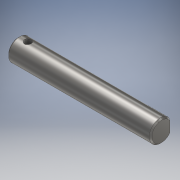
# Autodesk Inventor part: Crankshaft outer rod
Saved by Autodesk Inventor 2017 (Build 210142000, 142)
## iProperties
Created: 2018-11-11
Part Number: Crankshaft outer rod
Material: Steel, Alloy
Document SubType Name: Modeling
Designer: Arman Grewal
Density: 7.73 g/cm^3
Appearance: Semi-Polished
Author: Arman Grewal
Autodesk Inventor part; units mm, degrees
ref_plane "YZ Plane" through (0, 0, 0) normal (1, 0, 0) x (0, 1, 0)
ref_plane "XZ Plane" through (0, 0, 0) normal (0, 1, 0) x (-1, 0, 0)
sketch "Sketch1" plane through (0, 0, 0) normal (1, 0, 0) x (0, 1, 0)
  circle A0 centre (0, 0) radius 4
  dimension "d0" = 8
  constraints: 1 centre point, 1 coincident
  measures "d0" diameter of A0
extrude "Extrusion1" add sketch "Sketch1" along normal blind 52
chamfer "Chamfer1" distance 0.5 angle 45 2 edges at (0, -4, 0) (52, -4, 0)
ref_plane "Work Plane1" through (0, 0, 5.5) normal (0, 0, 1) x (1, 0, 0)
sketch "Sketch2" plane through (0, 0, 5.5) normal (0, 0, 1) x (1, 0, 0)
  line L0 (0, 0) -> (3.5, 0) construction
  circle A0 centre (3.5, 0) radius 1.25
  dimension "d7" = 3.5
  dimension "d8" = 2.5
  constraints: 2 end point, 1 centre point, 1 coincident, 1 horizontal
  measures "d7" distance of L0.start L0.end
  measures "d8" diameter of A0
extrude "Extrusion2" cut sketch "Sketch2" against normal blind 52
sketch "Sketch3" plane through (0, 0, 5.5) normal (0, 0, 1) x (1, 0, 0)
  line L0 (52, 3.5) -> (52, -3.5) construction
  line L1 (52, 0) -> (52, 3) construction
  line L2 (52, 3) -> (44, 3) construction
  line L3 (44, 3) -> (44, 4) construction
  line L4 (0.5, 4) -> (51.5, 4) construction
  line L5 (44, 4) -> (52, 4)
  line L6 (52, 4) -> (52, 3)
  line L7 (52, 3) -> (44, 3)
  line L8 (44, 3) -> (44, 4)
  point P0 (0, 0)
  dimension "d11" = 3
  dimension "d12" = 8
  constraints: 14 end point, 3 perpendicular, 2 parallel, 2 point on line, 1 horizontal, 1 midpoint
  measures "d11" distance of L1.start L1.end
  measures "d12" distance of L1.end L2.end
extrude "Extrusion3" cut sketch "Sketch3" against normal blind 52
body "Solid1"
